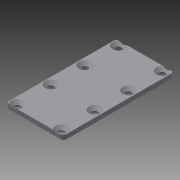
# Autodesk Inventor part: Tapa
Saved by Autodesk Inventor 2013 (Build 170138000, 138)
## iProperties
Created: 2014-06-18
Part Number: Tapa
Material: Genérico
Document SubType Name: Chapa
Designer: Administrador
Density: 1 g/cm^3
Sheet Metal Rule: Por defecto_mm
Author: Administrador
Autodesk Inventor part; units mm, degrees
ref_plane "YZ Plane" through (0, 0, 0) normal (1, 0, 0) x (0, 1, 0)
ref_plane "XZ Plane" through (0, 0, 0) normal (0, 1, 0) x (-1, 0, 0)
ref_plane "XY Plane" through (0, 0, 0) normal (0, 0, 1) x (1, 0, 0)
sketch "Boceto1" plane through (0, 0, 0) normal (0, 0, 1) x (1, 0, 0)
  circle A0 centre (-35.391, 9) radius 2
  circle A1 centre (-6.391, 31.3) radius 2
  circle A2 centre (-6.391, 75.8986) radius 2
  circle A3 centre (-35.391, 75.8986) radius 2
  circle A4 centre (-35.391, 53.6) radius 2
  circle A5 centre (-6.391, 53.6) radius 2
  circle A6 centre (-6.391, 9) radius 2
  circle A7 centre (-35.391, 31.3) radius 2
  line L0 (-39.891, 8) -> (-39.891, 77)
  arc A8 (-39.891, 8) -> (-37.891, 6) centre (-37.891, 8) ccw
  line L1 (-3.891, 6) -> (-37.891, 6)
  arc A9 (-3.891, 6) -> (-1.891, 8) centre (-3.891, 8) ccw
  line L2 (-1.891, 77) -> (-1.891, 8)
  arc A10 (-1.891, 77) -> (-3.891, 79) centre (-3.891, 77) ccw
  line L3 (-37.891, 79) -> (-3.891, 79)
  arc A11 (-37.891, 79) -> (-39.891, 77) centre (-37.891, 77) ccw
  point P0 (0, 0)
  point P1 (-20.891, 10)
  dimension "d0" = 38
  constraints: 12 centre point, 8 end point, 8 point on circle
  measures "d0" distance between parallel lines of L2 L0
extrude "Extrusión1" add sketch "Boceto1" along normal blind 3
sketch "Boceto2" plane through (0, 0, 3) normal (0, 0, 1) x (1, 0, 0)
  point P0 (0, 0)
  point P1 (-35.391, 75.8986)
  point P2 (-6.391, 75.8986)
  point P3 (-6.391, 53.6)
  point P4 (-35.391, 53.6)
  point P5 (-35.391, 31.3)
  point P6 (-6.391, 31.3)
  point P7 (-35.391, 9)
  point P8 (-6.391, 9)
hole "Hole2" at (-35.391, 75.8986, 3) at (-6.391, 75.8986, 3) at (-6.391, 53.6, 3) at (-35.391, 53.6, 3) at (-35.391, 31.3, 3) at (-6.391, 31.3, 3) at (-35.391, 9, 3) at (-6.391, 9, 3) direction (0, 0, -1) diameter 4 end through all countersink diameter 8 countersink angle 90
equation "\"d17\" = Grosor"
equation "\"Radio_pliegue\" = Grosor"
equation "\"Anchura_desahogo_plegado\" = Grosor"
equation "\"Profundidad_desahogo_plegado\" = 0.5 * Grosor"
equation "\"Tamaño_destalonado\" = 4 * Grosor"
equation "\"Remanente_mínimo\" = 2 * Grosor"
equation "\"Radiodetransición\" = Radio_pliegue"
equation "\"Tamaño_de_radio_de_Jacobi\" = Radio_pliegue"
equation "\"TamañoSeparación\" = Grosor"
equation "\"Grosor\" = 0.5"
